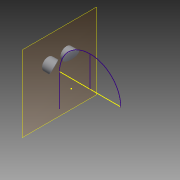
# Autodesk Inventor part: GhostEye
Saved by Autodesk Inventor 2015 (Build 190159000, 159)
## iProperties
Created: 2015-04-11
Part Number: GhostEye
Material: Generic
Document SubType Name: Modeling
Designer: tquinn
Density: 1 g/cm^3
Appearance: Default
Author: tquinn
Autodesk Inventor part; units mm, degrees
ref_plane "XZ Plane" through (0, 0, 0) normal (0, 1, 0) x (-1, 0, 0)
ref_plane "XY Plane" through (0, 0, 0) normal (0, 0, 1) x (1, 0, 0)
sketch "Sketch1" plane through (0, 0, 0) normal (0, 0, 1) x (1, 0, 0)
  arc A0 (20.3817, 3.6799) -> (-5.0183, 3.6799) centre (7.6817, 3.6799) ccw
  line L0 (-5.0183, -9.6551) -> (-5.0183, 3.6799)
  line L1 (-5.0183, 3.6799) -> (20.3817, 3.6799) projected
  line L2 (7.6817, 3.6799) -> (7.6817, 16.3799)
  point P0 (0, 0)
  constraints: 4 end point, 3 point on circle, 1 centre point, 1 vertical, 6 other
ref_plane "Work Plane1" through (-5.0183, 3.6799, 0) normal (1, 0, 0) x (0, 1, 0)
sketch "Sketch2" plane through (-5.0183, 3.6799, 0) normal (1, 0, 0) x (0, 1, 0)
  arc A0 (0, -12.7) -> (0, 12.7) centre (0, 0.8576) ccw
  line L0 (0, 12.7) -> (0, -12.7) projected
  line L1 (0, 12.7) -> (0, -12.7) projected
  circle A1 centre (5.08, 3.81) radius 2.54
  line L2 (12.671, 0) -> (-9.5008, 0)
  circle A2 centre (5.08, -3.81) radius 2.54
  point P0 (-3.6799, 0)
  dimension "d1" = 5.08
  dimension "d2" = 5.08
  dimension "d3" = 8.89
  constraints: 2 centre point, 2 end point, 1 perpendicular, 1 symmetric about line, 9 other
  measures "d1" diameter of A1
  measures "d2" distance from line of L0 A1.centre
  measures "d3" vertical distance of L0.start A1.centre
extrude "Extrusion1" add sketch "Sketch2" along normal blind 5.08 contours A1 | A2
sketch "Sketch3" plane through (0, 0, 0) normal (0, 0, 1) x (1, 0, 0)
  arc A0 (20.3817, 3.6799) -> (-5.0183, 3.6799) centre (7.6817, 3.6799) ccw projected
  line L0 (-5.0183, 3.6799) -> (20.3817, 3.6799) projected
  arc A1 (20.3817, 3.6799) -> (-5.0183, 3.6799) centre (7.6817, 3.6799) ccw
  line L1 (7.6817, 3.6799) -> (7.6817, 16.3799)
  arc A2 (7.6817, 16.3799) -> (-5.0183, 3.6799) centre (7.6817, 3.6799) ccw
  line L2 (7.6817, 3.6799) -> (-5.0183, 3.6799)
  line L3 (7.6817, 16.3799) -> (7.6817, 3.6799)
  circle A3 centre (7.6817, 3.6799) radius 13.208
  line L4 (7.6817, 3.6799) -> (-5.5263, 3.6799)
  line L5 (7.6817, 3.6799) -> (7.6817, 16.8879)
  arc A4 (7.6817, 16.8879) -> (-5.5263, 3.6799) centre (7.6817, 3.6799) ccw
  point P0 (0, 0)
  dimension "d7" = 0.508
  constraints: 10 end point, 9 point on circle, 4 centre point, 3 concentric, 2 collinear, 2 point on line, 1 coincident, 1 other
  measures "d7" radial gap between concentric circles of A0 A3
revolve "Revolution1" cut sketch "Sketch3" angle 360 about axis through (7.6817, 3.6799, 0) along (0, 1, 0) picked at (4.9029, 11.6212) contours L1 L0 A0
sketch "Sketch4" plane through (0, 0, 0) normal (0, 0, 1) x (1, 0, 0)
  arc A0 (20.3817, 3.6799) -> (-5.0183, 3.6799) centre (7.6817, 3.6799) ccw
  line L0 (7.6817, 3.6799) -> (7.6817, 16.3799)
  line L1 (7.6817, 3.6799) -> (-5.0183, 3.6799)
  circle A1 centre (7.6817, 3.6799) radius 13.081
  line L2 (7.6817, 16.7609) -> (7.6817, 3.6799)
  line L3 (7.6817, 3.6799) -> (-5.3993, 3.6799)
  arc A2 (7.6817, 16.7609) -> (-5.3993, 3.6799) centre (7.6817, 3.6799) ccw
  point P0 (0, 0)
  dimension "d8" = 0.381
  constraints: 8 end point, 7 point on circle, 3 centre point, 2 point on line, 1 coincident, 1 collinear, 1 concentric, 1 perpendicular, 4 other
  measures "d8" radial gap between concentric circles of A0 A1
revolve "Revolution2" cut sketch "Sketch4" angle 360 about axis through (7.6817, 16.7609, 0) along (0, -1, 0) keep common part contours A0 L3 A1 L2
body "Solid1"
